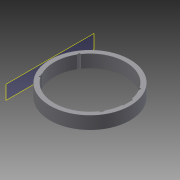
# Autodesk Inventor part: frame
Saved by Autodesk Inventor 2014 (Build 180170000, 170)
## iProperties
Created: 2013-05-24
Part Number: frame
Material: Generisch
Document SubType Name: Modeling
Designer: hartmann
Density: 1 g/cm^3
Appearance: Vorgabe
Author: hartmann
Autodesk Inventor part; units mm, degrees
ref_plane "YZ Plane" through (0, 0, 0) normal (1, 0, 0) x (0, 1, 0)
ref_plane "XZ Plane" through (0, 0, 0) normal (0, 1, 0) x (-1, 0, 0)
ref_plane "Arbeitsebene1" through (32.6, -4.2, 17.5) normal (0, 0, 1) x (1, 0, 0)
sketch "Skizze1" plane through (0, 0, 0) normal (0, 0, 1) x (1, 0, 0)
  circle A0 centre (0, 0) radius 49
  circle A1 centre (0, 0) radius 55
  circle A2 centre (-17, -10) radius 1.45 projected
  circle A3 centre (37.5, 15.5) radius 1.45 projected
  line L0 (-37.9, -24) -> (-42.5, -24) projected
  line L1 (-42.5, -24) -> (-42.5, -28) projected
  line L2 (-42.5, -28) -> (-7.5, -28) projected
  line L3 (-7.5, -28) -> (-7.5, -17.2) projected
  line L4 (-7.5, -17.2) -> (7.5, -17.2) projected
  line L5 (7.5, -17.2) -> (7.5, -28) projected
  line L6 (7.5, -28) -> (42.5, -28) projected
  line L7 (42.5, -28) -> (42.5, -26.8) projected
  line L8 (42.5, -26.8) -> (22.5, -26.8) projected
  line L9 (22.5, -26.8) -> (22.5, -10.8) projected
  line L10 (22.5, -10.8) -> (42.5, -10.8) projected
  line L11 (42.5, -10.8) -> (42.5, -4.2) projected
  line L12 (42.5, -4.2) -> (32.6, -4.2) projected
  line L13 (32.6, -4.2) -> (32.6, 9) projected
  line L14 (32.6, 9) -> (42.5, 9) projected
  line L15 (42.5, 9) -> (42.5, 28) projected
  line L16 (42.5, 28) -> (28, 28) projected
  line L17 (28, 28) -> (28, 16.5) projected
  line L18 (28, 16.5) -> (16, 16.5) projected
  line L19 (16, 16.5) -> (16, 28) projected
  line L20 (16, 28) -> (-42.5, 28) projected
  line L21 (-42.5, 28) -> (-42.5, -16.5) projected
  line L22 (-42.5, -16.5) -> (-37.9, -16.5) projected
  line L23 (-37.9, -16.5) -> (-37.9, -24) projected
  line L24 (-8.8, 27) -> (-8.8, 22) projected
  line L25 (-8.8, 22) -> (-41.5, 22) projected
  line L26 (-41.5, 22) -> (-41.5, 27) projected
  line L27 (-41.5, 27) -> (-8.8, 27) projected
  line L28 (-1.5, 15.5) -> (-1.5, 25.5) projected
  line L29 (-1.5, 25.5) -> (8.5, 25.5) projected
  line L30 (8.5, 25.5) -> (8.5, 15.5) projected
  line L31 (8.5, 15.5) -> (-1.5, 15.5) projected
  line L32 (43.5, -10.8) -> (22.5, -10.8) projected
  line L33 (22.5, -10.8) -> (22.5, -26.8) projected
  line L34 (22.5, -26.8) -> (43.5, -26.8) projected
  line L35 (43.5, -26.8) -> (43.5, -10.8) projected
  line L36 (32.6, -4.2) -> (50, -4.2) projected
  line L37 (50, -4.2) -> (50, 9) projected
  line L38 (50, 9) -> (32.6, 9) projected
  line L39 (32.6, 9) -> (32.6, -4.2) projected
  line L40 (-43.5, -24) -> (-37.9, -24) projected
  line L41 (-37.9, -24) -> (-37.9, -16.5) projected
  line L42 (-37.9, -16.5) -> (-43.5, -16.5) projected
  line L43 (-43.5, -16.5) -> (-43.5, -24) projected
  line L44 (43.5, -22.5555) -> (43.5, -26.8)
  line L45 (41.0215, -26.8) -> (43.5, -26.8)
  line L46 (42.5, -26.8) -> (42.5, -28)
  line L47 (40.2119, -28) -> (42.5, -28)
  line L48 (48.8197, -4.2) -> (50, -4.2)
  line L49 (50, -4.2) -> (50, 9)
  line L50 (50, 9) -> (48.1664, 9)
  line L51 (42.5, 24.3875) -> (42.5, 28)
  line L52 (42.5, 28) -> (40.2119, 28)
  line L53 (-42.5, 24.3875) -> (-42.5, 28)
  line L54 (-42.5, 28) -> (-40.2119, 28)
  line L55 (-40.2119, -28) -> (-42.5, -28)
  line L56 (-42.5, -28) -> (-42.5, -24.3875)
  line L57 (-42.72, -24) -> (-43.5, -24)
  line L58 (-43.5, -24) -> (-43.5, -22.5555)
  dimension "d1" = 110
  dimension "d2" = 6
  constraints: 30 end point, 13 point on line, 8 collinear, 2 coincident, 1 centre point, 1 parallel, 1 perpendicular, 15 other
  measures "d1" diameter of A1
extrude "Extrusion3" add sketch "Skizze1" along normal up to surface (17.5 mm away) contours A1
ref_plane "Work Plane3" through (-55, 0, 0) normal (-1, 0, 0) x (0, -1, 0)
ref_plane "Work Plane2" through (-26.6759, -34.6142, 17.5) normal (-1, 0, 0) x (0, 0, 1)
sketch "Sketch2" plane through (-55, 0, 0) normal (-1, 0, 0) x (0, -1, 0)
  line L0 (56.7996, 2.8291) -> (24.1561, 2.8291) construction
  line L1 (24.1561, 2.8291) -> (24.1561, 14.6895) construction
  line L2 (24.1561, 14.6895) -> (56.7996, 14.6895) construction
  line L3 (56.7996, 14.6895) -> (56.7996, 2.8291) construction
  spline S0 degree 2 poles (48.5615, 10.337) (48.5615, 11.3529) (49.4424, 12.091) knots 0 0 0 1 1 1
  spline S1 degree 2 poles (49.4424, 12.091) (50.3155, 12.8291) (51.5535, 12.8291) knots 0 0 0 1 1 1
  line L4 (51.5535, 12.8291) -> (56.0615, 12.8291)
  line L5 (56.0615, 12.8291) -> (56.0615, 2.8291)
  line L6 (56.0615, 2.8291) -> (51.5535, 2.8291)
  spline S2 degree 2 poles (51.5535, 2.8291) (50.3393, 2.8291) (49.4424, 3.5751) knots 0 0 0 1 1 1
  spline S3 degree 2 poles (49.4424, 3.5751) (48.5615, 4.3132) (48.5615, 5.337) knots 0 0 0 1 1 1
  line L7 (48.5615, 5.337) -> (48.5615, 5.464)
  spline S4 degree 2 poles (48.5615, 5.464) (48.5615, 6.2656) (49.1409, 6.9164) knots 0 0 0 1 1 1
  spline S5 degree 2 poles (49.1409, 6.9164) (49.4345, 7.2497) (50.1567, 7.7101) (50.6329, 7.8291) knots 0 0 0 1 2 2 2
  spline S6 degree 2 poles (50.6329, 7.8291) (50.1409, 7.964) (49.371, 8.4481) (48.8393, 9.1069) (48.5615, 9.9005) (48.5615, 10.337) knots 0 0 0 1 2 3 4 4 4
  spline S7 degree 2 poles (50.8075, 9.3847) (50.8075, 9.1942) (50.9821, 8.8608) (51.2916, 8.6148) (51.7043, 8.4561) (51.9345, 8.4561) knots 0 0 0 1 2 3 4 4 4
  line L8 (51.9345, 8.4561) -> (54.5535, 8.4561)
  line L9 (54.5535, 8.4561) -> (54.5535, 10.337)
  line L10 (54.5535, 10.337) -> (51.9345, 10.337)
  spline S8 degree 2 poles (51.9345, 10.337) (51.7043, 10.337) (51.2916, 10.1783) (50.9821, 9.9243) (50.8075, 9.5831) (50.8075, 9.3847) knots 0 0 0 1 2 3 4 4 4
  spline S9 degree 2 poles (50.8075, 6.2735) (50.8075, 6.0831) (50.9821, 5.7418) (51.2916, 5.4799) (51.7043, 5.337) (51.9345, 5.337) knots 0 0 0 1 2 3 4 4 4
  line L11 (51.9345, 5.337) -> (54.5535, 5.337)
  line L12 (54.5535, 5.337) -> (54.5535, 7.2021)
  line L13 (54.5535, 7.2021) -> (51.9345, 7.2021)
  spline S10 degree 2 poles (51.9345, 7.2021) (51.7043, 7.2021) (51.2916, 7.0593) (50.9821, 6.8053) (50.8075, 6.472) (50.8075, 6.2735) knots 0 0 0 1 2 3 4 4 4
  spline S11 degree 2 poles (44.0615, 12.8291) (45.3155, 12.8291) (46.1805, 12.1069) knots 0 0 0 1 1 1
  spline S12 degree 2 poles (46.1805, 12.1069) (46.625, 11.7339) (47.0694, 10.8529) (47.0694, 10.337) knots 0 0 0 1 2 2 2
  line L14 (47.0694, 10.337) -> (47.0694, 2.8291)
  line L15 (47.0694, 2.8291) -> (41.0694, 2.8291)
  line L16 (41.0694, 2.8291) -> (41.0694, 5.337)
  line L17 (41.0694, 5.337) -> (45.5615, 5.337)
  line L18 (45.5615, 5.337) -> (45.5615, 7.2021)
  line L19 (45.5615, 7.2021) -> (42.5615, 7.2021)
  line L20 (42.5615, 7.2021) -> (42.5615, 8.4561)
  line L21 (42.5615, 8.4561) -> (45.5615, 8.4561)
  line L22 (45.5615, 8.4561) -> (45.5615, 9.0831)
  spline S13 degree 2 poles (45.5615, 9.0831) (45.5615, 9.3529) (45.3313, 9.8053) (44.9266, 10.1386) (44.3789, 10.337) (44.0615, 10.337) knots 0 0 0 1 2 3 4 4 4
  line L23 (44.0615, 10.337) -> (41.0694, 10.337)
  line L24 (41.0694, 10.337) -> (41.0694, 12.8291)
  line L25 (41.0694, 12.8291) -> (44.0615, 12.8291)
  spline S14 degree 2 poles (36.5694, 12.8291) (37.8234, 12.8291) (38.6885, 12.1069) knots 0 0 0 1 1 1
  spline S15 degree 2 poles (38.6885, 12.1069) (39.1329, 11.7339) (39.5774, 10.8529) (39.5774, 10.337) knots 0 0 0 1 2 2 2
  line L26 (39.5774, 10.337) -> (39.5774, 2.8291)
  line L27 (39.5774, 2.8291) -> (33.5774, 2.8291)
  line L28 (33.5774, 2.8291) -> (33.5774, 5.337)
  line L29 (33.5774, 5.337) -> (38.0694, 5.337)
  line L30 (38.0694, 5.337) -> (38.0694, 7.2021)
  line L31 (38.0694, 7.2021) -> (35.0694, 7.2021)
  line L32 (35.0694, 7.2021) -> (35.0694, 8.4561)
  line L33 (35.0694, 8.4561) -> (38.0694, 8.4561)
  line L34 (38.0694, 8.4561) -> (38.0694, 9.0831)
  spline S16 degree 2 poles (38.0694, 9.0831) (38.0694, 9.3529) (37.8393, 9.8053) (37.4345, 10.1386) (36.8869, 10.337) (36.5694, 10.337) knots 0 0 0 1 2 3 4 4 4
  line L35 (36.5694, 10.337) -> (33.5774, 10.337)
  line L36 (33.5774, 10.337) -> (33.5774, 12.8291)
  line L37 (33.5774, 12.8291) -> (36.5694, 12.8291)
  spline S17 degree 2 poles (24.5853, 5.964) (24.5853, 6.9799) (25.4662, 7.718) knots 0 0 0 1 1 1
  spline S18 degree 2 poles (25.4662, 7.718) (25.9107, 8.0831) (26.9583, 8.4561) (27.5774, 8.4561) knots 0 0 0 1 2 2 2
  line L38 (27.5774, 8.4561) -> (30.5774, 8.4561)
  line L39 (30.5774, 8.4561) -> (30.5774, 12.8291)
  line L40 (30.5774, 12.8291) -> (32.0853, 12.8291)
  line L41 (32.0853, 12.8291) -> (32.0853, 2.8291)
  line L42 (32.0853, 2.8291) -> (27.5774, 2.8291)
  spline S19 degree 2 poles (27.5774, 2.8291) (26.3631, 2.8291) (25.4662, 3.5751) knots 0 0 0 1 1 1
  spline S20 degree 2 poles (25.4662, 3.5751) (24.5853, 4.3132) (24.5853, 5.337) knots 0 0 0 1 1 1
  line L43 (24.5853, 5.337) -> (24.5853, 5.964)
  spline S21 degree 2 poles (26.8313, 6.2735) (26.8313, 6.0831) (27.0059, 5.7418) (27.3155, 5.4799) (27.7282, 5.337) (27.9583, 5.337) knots 0 0 0 1 2 3 4 4 4
  line L44 (27.9583, 5.337) -> (30.5774, 5.337)
  line L45 (30.5774, 5.337) -> (30.5774, 7.2021)
  line L46 (30.5774, 7.2021) -> (27.9583, 7.2021)
  spline S22 degree 2 poles (27.9583, 7.2021) (27.7282, 7.2021) (27.3155, 7.0593) (27.0059, 6.8053) (26.8313, 6.472) (26.8313, 6.2735) knots 0 0 0 1 2 3 4 4 4
  point P0 (0, 0)
  constraints: 2 other
emboss "Prägen1" sketch "Sketch2" operation cut depth 3 direction (-1, 0, 0) wrap yes faces at (-50.386, -22.0512, 11.6667)
